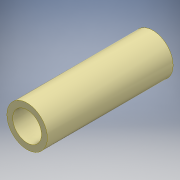
# Autodesk Inventor part: RPS Spacer
Saved by Autodesk Inventor 2016 (Build 200138000, 138)
## iProperties
Created: 2016-11-14
Part Number: RPS Spacer
Material: Nylon 6/6
Document SubType Name: Modeling
Designer: R.P. SMITH
Mass: 0.124374 g
Surface Area: 3.54387 cm^2
Volume: 0.110066 cm^3
Density: 1.13 g/cm^3
Appearance: Nylon 6
Author: R.P. SMITH
Autodesk Inventor part; units mm, degrees
ref_plane "YZ Plane" through (0, 0, 0) normal (1, 0, 0) x (0, 1, 0)
ref_plane "XZ Plane" through (0, 0, 0) normal (0, 1, 0) x (-1, 0, 0)
ref_plane "XY Plane" through (0, 0, 0) normal (0, 0, 1) x (1, 0, 0)
sketch "Sketch1" plane through (0, 0, 0) normal (0, 1, 0) x (-1, 0, 0)
  circle A0 centre (0, 0) radius 2.25
  circle A1 centre (0, 0) radius 1.6
  dimension "d0" = 4.5
  dimension "d1" = 3.2
  constraints: 2 centre point, 2 coincident
  measures "d0" diameter of A0
  measures "d1" diameter of A1
extrude "Extrusion1" add sketch "Sketch1" along normal mid plane 14
body "Solid1"
